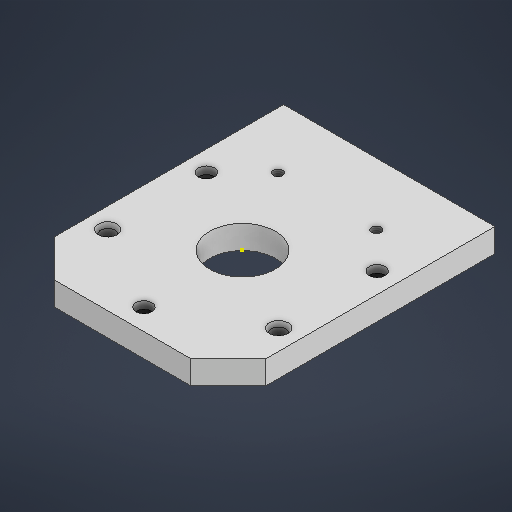
# Autodesk Inventor part: encoder mount
Saved by Autodesk Inventor 2025.2 (Build 292293000, 293)
## iProperties
Created: 2025-06-02
Part Number: encoder mount
Material: Generic
Document SubType Name: Modeling
Designer: klawy
Density: 1 g/cm^3
Appearance: Default
Author: klawy
Autodesk Inventor part; units mm, degrees
ref_plane "YZ Plane" through (0, 0, 0) normal (1, 0, 0) x (0, 1, 0)
ref_plane "XZ Plane" through (0, 0, 0) normal (0, 1, 0) x (-1, 0, 0)
ref_plane "XY Plane" through (0, 0, 0) normal (0, 0, 1) x (1, 0, 0)
sketch "Sketch1" plane through (0, 0, 0) normal (0, 1, 0) x (-1, 0, 0)
  line L0 (-22.5, 28.5) -> (22.5, 28.5)
  line L1 (22.5, 28.5) -> (22.5, -28.5)
  line L2 (22.5, -28.5) -> (-22.5, -28.5)
  line L3 (-22.5, -28.5) -> (-22.5, 28.5)
  line L4 (-22.5, 28.5) -> (22.5, -28.5) construction
  line L5 (22.5, 28.5) -> (-22.5, -28.5) construction
  circle A0 centre (0, 0) radius 21 construction
  line L6 (0, -43.2) -> (0, 40.45) projected
  line L7 (22.5, -28.5) -> (-22.5, -28.5)
  line L8 (-22.5, -28.5) -> (-22.5, -31.25)
  line L9 (-22.5, -31.25) -> (22.5, -31.25)
  line L10 (22.5, -31.25) -> (22.5, -28.5)
  point P0 (0, 21)
  point P1 (-18.1865, -10.5)
  point P2 (18.1865, -10.5)
  dimension "d2" = 42
  dimension "d0" = 45
  dimension "d1" = 57
  dimension "d5" = 360
  dimension "d62" = 2.75
  constraints: 20 end point, 4 parallel, 2 horizontal, 2 midpoint, 2 perpendicular, 2 point on line, 1 coincident, 1 vertical alignment, 6 other
  measures "d0" distance of L0.start L0.end
  measures "d1" distance of L0.end L1.end
  measures "d62" distance between parallel lines of L2 L9
extrude "Extrusion1" add sketch "Sketch1" along normal blind 5
hole "Hole1" at (0, 0, 21) at (18.1865, 0, -10.5) at (-18.1865, 0, -10.5) direction (0, 1, 0) diameter 3.4 depth 8.8 tip angle 118 counterbore diameter 6.5 counterbore depth 3.4 clearance for "Socket Head Cap Screw ISO 4762" size "M3" standard "ISO"
sketch "Sketch2" plane through (0, 0, 0) normal (0, -1, 0) x (1, 0, 0)
  circle A0 centre (0, 0) radius 7
  dimension "d16" = 14
  constraints: 1 centre point, 1 coincident
  measures "d16" diameter of A0
extrude "Extrusion2" cut sketch "Sketch2" against normal through all
sketch "Sketch3" plane through (0, 5, 0) normal (0, 1, 0) x (1, 0, 0)
  circle A0 centre (0, 0) radius 21 construction
  point P0 (18.1865, -10.5)
  point P1 (0, 21)
  point P2 (-18.1865, -10.5)
  dimension "d19" = 42
  dimension "d22" = 360
  constraints: 1 coincident, 7 other
hole "Hole2" at (18.1865, 5, 10.5) at (-18.1865, 5, 10.5) direction (0, -1, 0) diameter 3 depth 8.8 tip angle 118
chamfer "Chamfer1" distance 0.5 angle 60 2 edges at (-18.1865, 5, 9) (18.1865, 5, 9) measured on face at (-0.2813, 5, -23.1497)
sketch "Sketch5" plane through (0, 0, 0) normal (0, -1, 0) x (1, 0, 0)
  line L0 (-13.3095, -20.83) -> (13.6905, -20.83)
  line L1 (13.6905, -20.83) -> (13.6905, -8.83)
  line L2 (13.6905, -8.83) -> (-13.3095, -8.83)
  line L3 (-13.3095, -8.83) -> (-13.3095, -20.83)
  line L4 (-13.3095, -20.83) -> (13.6905, -8.83) construction
  line L5 (13.6905, -20.83) -> (-13.3095, -8.83) construction
  line L6 (0, -36.4441) -> (0, 10.0043) construction
  circle A0 centre (0, 0) radius 7 projected
  point P0 (0.1905, -14.83)
  point P1 (3.4689, -6.08)
  point P2 (-3.4689, -6.08)
  dimension "d34" = 12
  dimension "d35" = 27
  dimension "d36" = 13.3095
  dimension "d38" = 20.83
  constraints: 14 end point, 2 midpoint, 2 parallel, 1 horizontal, 1 perpendicular, 1 point on line, 1 vertical
  measures "d34" distance of L0.end L1.end
  measures "d35" distance between parallel lines of L1 L3
  measures "d36" distance between parallel lines of L6 L3
  measures "d38" distance from line of A0.centre L0
extrude "Extrusion3" cut sketch "Sketch5" against normal blind 1 contours L3 L2 L1 L0
sketch "Sketch6" plane through (0, 1, 0) normal (0, -1, 0) x (1, 0, 0)
  circle A0 centre (-10.4775, -18.036) radius 1.1414 construction
  line L0 (-13.3095, -20.83) -> (-13.3095, -8.83) projected
  line L1 (13.6905, -20.83) -> (-13.3095, -20.83) projected
  circle A1 centre (10.4775, -18.036) radius 1.164 construction
  line L2 (-10.4775, -18.036) -> (12.0154, -18.036) construction
  point P0 (0, 0)
  dimension "d41" = 2.832
  dimension "d42" = 2.794
  dimension "d43" = 20.955
  constraints: 2 centre point, 2 coincident, 2 end point, 1 horizontal, 1 point on line
  measures "d41" distance from line of L0 L2.start
  measures "d42" distance from line of L1 L2.start
  measures "d43" distance of A1.centre L2.start
hole "Hole3" at (10.4775, 1, -18.036) at (-10.4775, 1, -18.036) direction (0, 1, 0) diameter 2.013 depth 7.6 tip angle 118 thread size "M2.5x0.45" class "6H" standard "ISO Metric profile"
sketch "Sketch7" plane through (0, 0, 0) normal (0, -1, 0) x (1, 0, 0)
  line L0 (13.6905, -20.83) -> (-13.3095, -20.83) projected
  circle A0 centre (-11.3095, -20.83) radius 2
  line L1 (-13.3095, -20.83) -> (-13.3095, -8.83) projected
  line L2 (-9.3095, -20.83) -> (-9.3095, -23.83)
  line L3 (-13.3095, -20.83) -> (-13.3095, -23.83)
  line L4 (-9.3095, -23.83) -> (-13.3095, -23.83)
  line L5 (22.5, -31.25) -> (-22.5, -31.25) projected
  point P0 (0, 0)
  point P1 (-9.3095, -18.08)
  point P2 (-13.3095, -20.83)
  dimension "d51" = 4
  dimension "d63" = 3
  constraints: 6 end point, 3 vertical, 2 point on line, 3 other
  measures "d63" distance between parallel lines of L4 L0
extrude "Extrusion4" cut sketch "Sketch7" against normal blind 1
sketch "Sketch8" plane through (-22.5, 0, 28.5) normal (0, 0, 1) x (1, 0, 0)
  line L0 (25.75, 3.4) -> (19.25, 3.4) projected
  line L1 (0, 0) -> (45, 0) projected
  line L2 (45, 0) -> (45, 5) projected
  line L3 (0, 5) -> (45, 5) projected
  line L4 (0, 0) -> (0, 5) projected
  point P0 (22.5, 0)
extrude "Extrusion5" cut sketch "Sketch8" against normal blind 3
fillet "Fillet1" radius 2 5 edges at (13.6905, 0.5, -20.83) (13.6905, 0.5, -8.83) (-13.3095, 0.5, -8.83) (-9.3095, 0.5, -23.83) (-13.3095, 0.5, -23.83)
sketch "Sketch11" plane through (0, 5, 0) normal (0, 1, 0) x (1, 0, 0)
  point P0 (0, 0)
chamfer "Chamfer3" distance 8 angle 45 2 edges at (22.5, 2.5, 25.5) (-22.5, 2.5, 25.5)
body "Solid1"
